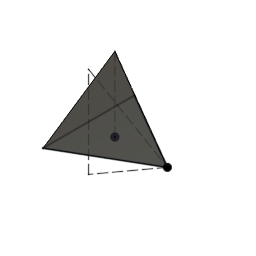
A3_AI22BTECH11005_2 (Autodesk Fusion 360 design; units mm, degrees)
Autodesk Fusion 360 part; units mm, degrees
sketch "Sketch1" plane through (0, 0, 0) normal (0, 1, 0) x (1, 0, 0)
  line L0 (-20.2073, 35) -> (-20.2073, -35) construction
  line L1 (-20.2073, -35) -> (40.4145, 0) construction
  line L2 (40.4145, 0) -> (-20.2073, 35) construction
  line L3 (40.4145, 0) -> (0, -57.1548) construction
  line L4 (0, -57.1548) -> (0, 0) construction
  dimension "d2" = 70
  constraint coincident L4.end origin
  constraint vertical L0
  constraint vertical L4
  constraint equal L1 L3
  measures "d2" distance of L1.end L3.end
sketch "Sketch2" plane through (0, 0, 0) normal (0, 0, 1) x (1, 0, 0)
  line L0 (40.4145, 0) -> (-20.2073, 35)
  line L1 (-20.2073, 35) -> (-20.2073, -35)
  line L2 (-20.2073, -35) -> (40.4145, 0)
  point P0 (40.4145, 0)
  constraint coincident P0 L0.start
loft "Loft1" add profiles "Sketch2" section 1 section 2 point at (0, 0, 57.1548)
